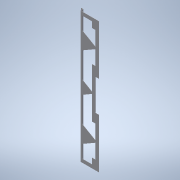
# Autodesk Inventor part: SP56V1 Chapa Detectores
Saved by Autodesk Inventor 2021.2 (Build 252289000, 289)
## iProperties
Created: 2026-10-05
Part Number: SP56V1 Chapa Detectores
Material: Stainless Steel AISI 430
Document SubType Name: Sheet Metal
Designer: nelso
Density: 7.85483 g/cm^3
Sheet Metal Rule: DD 1.56mm
Appearance: White
Author: nelso
Autodesk Inventor part; units mm, degrees
ref_plane "YZ Plane" through (0, 0, 0) normal (1, 0, 0) x (0, 1, 0)
ref_plane "XZ Plane" through (0, 0, 0) normal (0, 1, 0) x (-1, 0, 0)
ref_plane "XY Plane" through (0, 0, 0) normal (0, 0, 1) x (1, 0, 0)
sketch "Sketch1" plane through (0, 0, 0) normal (0, 1, 0) x (-1, 0, 0)
  line L0 (-30, 565) -> (30, 565) construction
  line L1 (30, 565) -> (30, -565) construction
  line L2 (30, -565) -> (-30, -565) construction
  line L3 (-30, -565) -> (-30, 565) construction
  line L4 (-30, 565) -> (30, -565) construction
  line L5 (30, 565) -> (-30, -565) construction
  line L6 (30, -565) -> (0, -565)
  line L7 (0, -565) -> (0, -485)
  line L8 (0, -485) -> (30, -485)
  line L9 (30, -485) -> (30, -565)
  line L10 (-30, -565) -> (0, -565)
  line L11 (0, -565) -> (0, -135)
  line L12 (0, -135) -> (-30, -135)
  line L13 (-30, -135) -> (-30, -565)
  line L14 (30, -135) -> (30, -215)
  line L15 (30, -215) -> (0, -215)
  line L16 (0, -215) -> (0, 215)
  line L17 (0, 215) -> (30, 215)
  line L18 (30, 215) -> (30, -215)
  line L19 (-30, 565) -> (0, 565)
  line L20 (0, 565) -> (0, 135)
  line L21 (0, 135) -> (-30, 135)
  line L22 (-30, 135) -> (-30, 565)
  line L23 (30, 565) -> (0, 565)
  line L24 (0, 565) -> (0, 485)
  line L25 (0, 485) -> (30, 485)
  line L26 (30, 485) -> (30, 565)
  point P0 (0, 0)
  dimension "d0" = 60
  dimension "d1" = 1130
  dimension "d2" = 80
  dimension "d3" = 430
  dimension "d4" = 80
  dimension "d5" = 430
  dimension "d6" = 430
  dimension "d7" = 80
  measures "d0" distance of L1.end L2.end
  measures "d1" distance of L0.end L1.end
  measures "d2" distance of L6.end L7.end
  measures "d3" distance of L11.end L10.end
  measures "d4" distance of L14.start L14.end
  measures "d5" distance of L15.end L16.end
  measures "d6" distance of L19.end L20.end
  measures "d7" distance of L24.end L23.end
sketch "Sketch2" plane through (0, 0, 0) normal (0, -1, 0) x (1, 0, 0)
  line L0 (-30, 485) -> (-30, 565)
  line L1 (-30, 565) -> (-130, 565)
  line L2 (-130, 565) -> (-130, 535)
  line L3 (-130, 535) -> (-30, 535)
  line L4 (-30, 535) -> (-30, 565)
  line L5 (-30, -485) -> (-30, -565)
  line L6 (-30, -565) -> (-130, -565)
  line L7 (-130, -565) -> (-130, -535)
  line L8 (-130, -535) -> (-30, -535)
  line L9 (-30, -535) -> (-30, -565)
  line L10 (-130, 565) -> (-130, -565)
  line L11 (0, 485) -> (0, 215)
  line L12 (0, 350) -> (15, 350)
  line L13 (-30, 215) -> (-30, -215)
  line L14 (-30, 0) -> (-15, 0)
  line L15 (0, -485) -> (0, -215)
  line L16 (0, -350) -> (15, -350)
  line L17 (15, 350) -> (-130, 266.2842)
  line L18 (-130, 433.7158) -> (15, 350)
  line L19 (-15, 0) -> (-130, -66.3953)
  line L20 (-130, 66.3953) -> (-15, 0)
  line L21 (15, -350) -> (-130, -433.7158)
  line L22 (-130, -266.2842) -> (15, -350)
  line L23 (-130, -565) -> (-115, -565)
  line L24 (-115, -565) -> (-115, 565)
  line L25 (-115, 565) -> (-130, 565)
  line L26 (-130, 565) -> (-130, -565)
  point P0 (0, 0)
  point P1 (-130, 350)
  point P2 (-130, 0)
  point P3 (-130, -350)
  dimension "d9" = 100
  dimension "d10" = 30
  dimension "d11" = 100
  dimension "d12" = 30
  dimension "d13" = 15
  dimension "d14" = 15
  dimension "d15" = 15
  dimension "d16" = 15
  measures "d9" distance of L3.end L2.end
  measures "d10" distance of L2.end L1.end
  measures "d11" distance of L7.end L8.end
  measures "d12" distance of L6.end L7.end
  measures "d13" distance of L12.start L12.end
  measures "d14" distance of L14.start L14.end
  measures "d15" distance of L16.start L16.end
  measures "d16" distance of L25.end L24.end
extrude "Plate1" add sketch "Sketch1" along normal blind 1.56
sheet face with bend "Face2" sketch "Sketch2" thickness 1.56 toward (0, 1, 0) bend radius 1.212 relief straight relief width 1.56 relief depth 0.78
bend "Bend1"
sketch "Sketch3" plane through (-128.44, 0, 565) normal (-1, 0, 0) x (0, -1, 0)
  line L0 (0, -1130) -> (0, 0)
  line L1 (0, 0) -> (-25, 0)
  line L2 (-25, 0) -> (-25, -1130)
  line L3 (-25, -1130) -> (0, -1130)
  constraints: 6 end point, 1 horizontal, 1 perpendicular, 1 vertical
edge flange "Flange1" height 25 angle 90 thickness 1.56 bend radius 1.212 thickness toward (-1, 0, 0) relief straight relief width 1.56 relief depth 0.78 edges at (-130, 1.56, 0) wall of the first edge with corners at (-128.44, 0, -565) (-128.44, 0, 565) (-128.44, 25, 565) (-128.44, 25, -565)
bend "Bend2"
corner "Corner1"
sketch "Sketch4" plane through (-128.44, 23.44, -565) normal (0, 1, 0) x (-1, 0, 0)
  line L0 (0, 1130) -> (0, 0)
  line L1 (0, 0) -> (20, 0)
  line L2 (20, 0) -> (20, 1130)
  line L3 (20, 1130) -> (0, 1130)
  constraints: 6 end point, 1 horizontal, 1 perpendicular, 1 vertical
edge flange "Flange2" height 20 angle 90 thickness 1.56 bend radius 1.212 thickness toward (0, 1, 0) relief straight relief width 1.56 relief depth 0.78 edges at (-130, 25, 0) wall of the first edge with corners at (-128.44, 23.44, 565) (-128.44, 23.44, -565) (-148.44, 23.44, -565) (-148.44, 23.44, 565)
bend "Bend3"
corner "Corner2"
equation "\"d8\" = Thickness"
equation "\"d17\" = BendRadius"
equation "\"d18\" = BendReliefWidth"
equation "\"d20\" = MinimumRemnant"
equation "\"d19\" = BendReliefDepth"
equation "\"d21\" = TransitionRadius"
equation "\"d22\" = BendReliefWidth"
equation "\"d23\" = BendReliefDepth"
equation "\"d24\" = MinimumRemnant"
equation "\"d25\" = TransitionRadius"
equation "\"d28\" = BendRadius"
equation "\"d29\" = CornerReliefSize"
equation "\"d30\" = GapSize"
equation "\"d31\" = JacobiRadiusSize"
equation "\"d32\" = BendReliefWidth"
equation "\"d33\" = BendReliefDepth"
equation "\"d34\" = MinimumRemnant"
equation "\"d35\" = TransitionRadius"
equation "\"d38\" = BendRadius"
equation "\"d39\" = CornerReliefSize"
equation "\"d40\" = GapSize"
equation "\"d41\" = JacobiRadiusSize"
equation "\"BendReliefWidth\" = Thickness"
equation "\"BendReliefDepth\" = 0.5 * Thickness"
equation "\"CornerReliefSize\" = 4 * Thickness"
equation "\"MinimumRemnant\" = 2 * Thickness"
equation "\"TransitionRadius\" = BendRadius"
equation "\"JacobiRadiusSize\" = BendRadius"
equation "\"GapSize\" = Thickness"
equation "\"Thickness\" = 1.56"
equation "\"BendRadius\" = 1.212"
body "Solid1"
